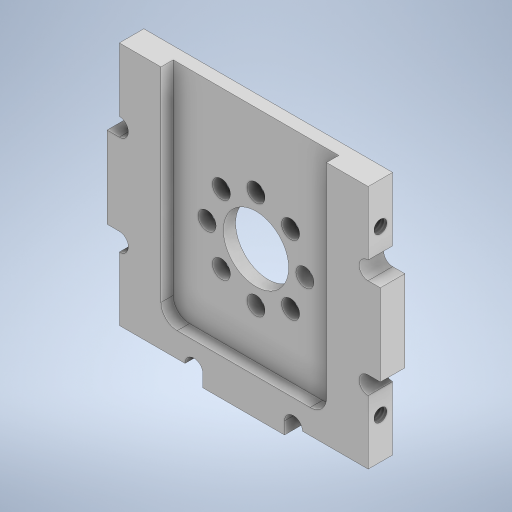
# Autodesk Inventor part: matarouru
Saved by Autodesk Inventor 2024 (Build 280153000, 153)
## iProperties
Created: 2024-06-06
Part Number: matarouru
Material: 一般
Document SubType Name: Modeling
Designer: right
Density: 1 g/cm^3
Appearance: 既定
Author: right
Autodesk Inventor part; units mm, degrees
ref_plane "YZ Plane" through (0, 0, 0) normal (1, 0, 0) x (0, 1, 0)
ref_plane "XZ Plane" through (0, 0, 0) normal (0, 1, 0) x (-1, 0, 0)
ref_plane "XY Plane" through (0, 0, 0) normal (0, 0, 1) x (1, 0, 0)
sketch "スケッチ1" plane through (0, 0, 0) normal (0, 0, 1) x (1, 0, 0)
  line L0 (-15.25, 15) -> (15.25, 15)
  line L1 (15.25, 15) -> (15.25, -15)
  line L2 (15.25, -15) -> (-15.25, -15)
  line L3 (-15.25, -15) -> (-15.25, 15)
  line L4 (-15.25, 15) -> (15.25, -15) construction
  line L5 (15.25, 15) -> (-15.25, -15) construction
  line L6 (-16.75, -5) -> (16.75, -5)
  line L7 (16.75, -5) -> (16.75, 5)
  line L8 (16.75, 5) -> (-16.75, 5)
  line L9 (-16.75, 5) -> (-16.75, -5)
  line L10 (-16.75, -5) -> (16.75, 5) construction
  line L11 (16.75, -5) -> (-16.75, 5) construction
  circle A0 centre (-15.25, 6.1) radius 1.1
  line L12 (0, 15) -> (0, 0) construction
  line L13 (-16.75, 0) -> (0, 0) construction
  circle A1 centre (15.25, 6.1) radius 1.1
  circle A2 centre (-15.25, -6.1) radius 1.1
  circle A3 centre (15.25, -6.1) radius 1.1
  point P0 (-15.25, -5)
  point P1 (-15.25, -7.2)
  point P2 (15.25, -7.2)
  point P3 (15.25, -5)
  point P4 (15.25, 5)
  point P5 (15.25, 7.2)
  point P6 (-15.25, 7.2)
  point P7 (-15.25, 5)
  dimension "d0" = 1.5
  dimension "d1" = 10
  dimension "d2" = 30.5
  dimension "d3" = 30
  dimension "d4" = 2.2
  constraints: 28 end point, 6 midpoint, 4 centre point, 4 parallel, 3 perpendicular, 3 symmetric about line, 2 horizontal, 1 point on line, 1 tangent, 1 vertical, 3 other
  measures "d0" distance between parallel lines of L1 L7
  measures "d1" distance of L6.end L7.end
  measures "d2" distance of L0.start L0.end
  measures "d3" distance of L2.end L0.start
  measures "d4" diameter of A0
extrude "押し出し1" add sketch "スケッチ1" along normal blind 3 contours L0 L1 A1 L8 A0 L3 | L8 L1 L6 L3 | L3 L6 L9 L8 | L8 L7 L6 L1 | L6 A3 L1 L2 L3 A2
sketch "スケッチ2" plane through (15.25, -15, 0) normal (1, 0, 0) x (0, 0, -1)
  line L0 (0, 7.8) -> (-3, 7.8) projected
  line L1 (0, 10) -> (-3, 10) projected
  line L2 (0, 20) -> (-3, 20) projected
  point P0 (0, 15)
  point P1 (-1.5, 5)
  point P2 (-1.5, 25)
  point P3 (-1.5, 7.8)
  dimension "d7" = 5
  dimension "d8" = 5
  constraints: 2 vertical alignment, 1 midpoint
  measures "d7" distance from line of L1 point (-1.5, 5)
  measures "d8" distance from line of L2 point (-1.5, 25)
hole "穴1" at (15.25, -10, 1.5) at (15.25, 10, 1.5) direction (-1, 0, 0) diameter 1.567 depth 4 tip angle 118 thread size "M2x0.4" class "6H" standard "ISO Metric profile"
sketch "スケッチ3" plane through (0, 0, 3) normal (0, 0, 1) x (1, 0, 0)
  circle A0 centre (0, 0) radius 4
  circle A1 centre (0, 0) radius 6 construction
  circle A2 centre (0, 6) radius 1.1
  circle A3 centre (-4.2426, 4.2426) radius 1.1
  circle A4 centre (-6, 0) radius 1.1
  circle A5 centre (-4.2426, -4.2426) radius 1.1
  circle A6 centre (0, -6) radius 1.1
  circle A7 centre (4.2426, -4.2426) radius 1.1
  circle A8 centre (6, 0) radius 1.1
  circle A9 centre (4.2426, 4.2426) radius 1.1
  dimension "d17" = 12
  dimension "d16" = 8
  dimension "d18" = 2.2
  dimension "d21" = 360
  constraints: 9 centre point, 2 coincident, 2 vertical alignment, 19 other
  measures "d16" diameter of A0
  measures "d18" diameter of A2
extrude "押し出し2" cut sketch "スケッチ3" against normal through all
sketch "スケッチ4" plane through (0, 0, 3) normal (0, 0, 1) x (1, 0, 0)
  line L0 (-10.15, -15) -> (10.15, -15)
  line L1 (10.15, -15) -> (10.15, 15)
  line L2 (10.15, 15) -> (-10.15, 15)
  line L3 (-10.15, 15) -> (-10.15, -15)
  line L4 (-10.15, -15) -> (10.15, 15) construction
  line L5 (10.15, -15) -> (-10.15, 15) construction
  arc A0 (15.25, 7.2) -> (15.25, 5) centre (15.25, 6.1) ccw projected
  line L6 (15.25, 15) -> (-15.25, 15) projected
  line L7 (10.15, -12) -> (-10.15, -12)
  line L8 (-5, -15) -> (5, -15)
  line L9 (5, -15) -> (5, -16.5)
  line L10 (5, -16.5) -> (-5, -16.5)
  line L11 (-5, -16.5) -> (-5, -15)
  circle A1 centre (-6.1, -15) radius 1.1
  circle A2 centre (6.1, -15) radius 1.1
  point P0 (0, 0)
  point P1 (14.15, 6.1)
  point P2 (0, -16.5)
  point P3 (0, -15)
  point P4 (-7.2, -15)
  point P5 (7.2, -15)
  dimension "d37" = 2.2
  dimension "d25" = 4
  dimension "d35" = 10
  dimension "d36" = 1.5
  dimension "d38" = 3
  constraints: 22 end point, 6 point on line, 4 midpoint, 4 parallel, 3 perpendicular, 2 horizontal, 1 point on circle, 1 vertical alignment, 6 other
  measures "d25" distance from line of point (14.15, 6.1) L1
  measures "d35" distance of L9.end L10.end
  measures "d36" distance between parallel lines of L8 L10
  measures "d38" distance between parallel lines of L0 L7
extrude "押し出し3" cut sketch "スケッチ4" against normal blind 1.5 contours L0 A1 | A2 L0 | L3 L2 L1 L7 picked at (-6.0558, -14.636) picked at (6.1442, -14.636)
sketch "スケッチ5" plane through (-15.25, 7.2, 0) normal (-1, 0, 0) x (0, 0, 1)
  line L0 (3, 0) -> (3, 7.8) projected
  circle A0 centre (1.5, 2.8) radius 0.7835 projected
  circle A1 centre (1.5, -17.2) radius 0.7835 projected
  point P0 (0, -7.2)
  constraints: 2 coincident
hole "穴2" at (-15.25, 10, 1.5) at (-15.25, -10, 1.5) direction (1, 0, 0) diameter 1.567 depth 4 tip angle 118 thread size "M2x0.4" class "6H" standard "ISO Metric profile"
extrude "押し出し4" add sketch "スケッチ4" against normal up to surface (3 mm away) contours L0 L9 L10 L11
extrude "押し出し5" cut sketch "スケッチ4" against normal through all contours L0 A1 | A2 L0 picked at (-6.0558, -14.636) picked at (6.1442, -14.636)
fillet "フィレット1" radius 2 2 edges at (-10.15, -12, 2.25) (10.15, -12, 2.25)
equation "\"d8\" = d7"
